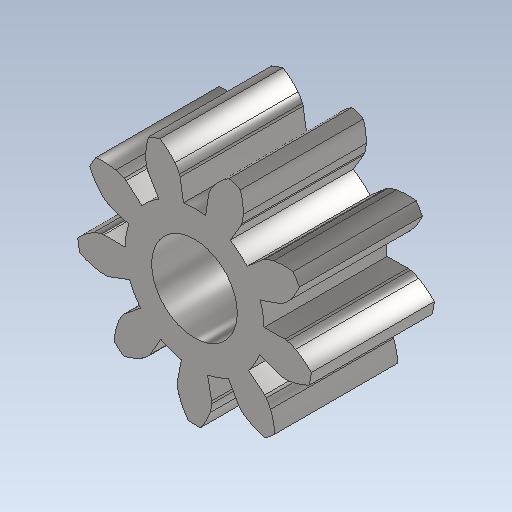
# Autodesk Inventor part: m1歯数9ギアd4t5
Saved by Autodesk Inventor 2020.2 (Build 242310000, 310)
## iProperties
Created: 2020-03-15
Part Number: m1歯数9ギアd4t5
Material: 鋼、炭素鋼
Document SubType Name: Modeling
Designer: aoyam
Density: 7.85 g/cm^3
Appearance: 半つや出し
Mass: 2.14409 g
Surface Area: 5.02952 cm^2
Volume: 0.273133 cm^3
Author: aoyam
Autodesk Inventor part; units mm, degrees
ref_plane "YZ Plane" through (0, 0, 0) normal (1, 0, 0) x (0, 1, 0)
ref_plane "XZ Plane" through (0, 0, 0) normal (0, 1, 0) x (-1, 0, 0)
ref_plane "XY Plane" through (0, 0, 0) normal (0, 0, 1) x (1, 0, 0)
sketch "スケッチ1" plane through (0, 0, 0) normal (0, 0, 1) x (1, 0, 0)
  arc A0 (1.9666, 4.772) -> (1.9302, 4.6607) centre (2.4755, 4.5436) ccw
  arc A1 (2.1768, 5.1207) -> (1.9666, 4.772) centre (3.3978, 4.1472) ccw
  arc A2 (2.8705, 5.7442) -> (2.1768, 5.1207) centre (4.3759, 3.3715) ccw
  arc A3 (0.5859, 4.6607) -> (0.5494, 4.772) centre (0.0406, 4.5436) ccw
  arc A4 (0.5494, 4.772) -> (0.3392, 5.1207) centre (-0.8817, 4.1472) ccw
  arc A5 (0.3392, 5.1207) -> (-0.3545, 5.7442) centre (-1.8598, 3.3715) ccw
  arc A6 (1.7746, 3.6946) -> (0.7414, 3.6946) centre (1.258, 0.4859) ccw
  arc A7 (-0.3545, 5.7442) -> (-0.8867, 5.5505) centre (1.258, 0.4859) ccw
  line L0 (1.7746, 3.6946) -> (1.9302, 4.6607)
  line L1 (0.7414, 3.6946) -> (0.5859, 4.6607)
  line L2 (-1.2002, 2.6118) -> (-1.9404, 3.2519)
  arc A8 (-1.9404, 3.2519) -> (-2.0398, 3.3137) centre (-2.2829, 2.8117) ccw
  arc A9 (-2.0398, 3.3137) -> (-2.425, 3.4458) centre (-2.7345, 1.9152) ccw
  arc A10 (-2.425, 3.4458) -> (-3.3572, 3.4775) centre (-2.9852, 0.6922) ccw
  arc A11 (-3.3572, 3.4775) -> (-3.6404, 2.987) centre (1.258, 0.4859) ccw
  arc A12 (-0.4087, 3.2759) -> (-1.2002, 2.6118) centre (1.258, 0.4859) ccw
  arc A13 (-0.9542, 4.2247) -> (-0.9106, 4.116) centre (-0.4176, 4.3769) ccw
  line L3 (-0.4087, 3.2759) -> (-0.9106, 4.116)
  arc A14 (-1.0174, 4.627) -> (-0.9542, 4.2247) centre (0.5437, 4.666) ccw
  arc A15 (-0.8867, 5.5505) -> (-1.0174, 4.627) centre (1.7917, 4.7005) ccw
  line L4 (-1.9916, 0.5343) -> (-2.9701, 0.5489)
  arc A16 (-2.9701, 0.5489) -> (-3.086, 0.5323) centre (-2.9495, -0.0085) ccw
  arc A17 (-3.086, 0.5323) -> (-3.466, 0.3859) centre (-2.7192, -0.9856) ccw
  arc A18 (-3.466, 0.3859) -> (-4.2004, -0.189) centre (-2.1251, -2.0836) ccw
  arc A19 (-4.2004, -0.189) -> (-4.102, -0.7468) centre (1.258, 0.4859) ccw
  arc A20 (-1.8122, 1.5518) -> (-1.9916, 0.5343) centre (1.258, 0.4859) ccw
  arc A21 (-2.8399, 1.928) -> (-2.7367, 1.8728) centre (-2.5267, 2.3895) ccw
  line L5 (-1.8122, 1.5518) -> (-2.7367, 1.8728)
  arc A22 (-3.1469, 2.1955) -> (-2.8399, 1.928) centre (-1.9761, 3.2289) ccw
  arc A23 (-3.6404, 2.987) -> (-3.1469, 2.1955) centre (-1.0423, 4.0575) ccw
  line L6 (-1.2625, -1.5659) -> (-2.0214, -2.1837)
  arc A24 (-2.0214, -2.1837) -> (-2.0995, -2.2708) centre (-1.6474, -2.5974) ccw
  arc A25 (-2.0995, -2.2708) -> (-2.2965, -2.6273) centre (-0.8429, -3.1978) ccw
  arc A26 (-2.2965, -2.6273) -> (-2.4895, -3.5398) centre (0.318, -3.6571) ccw
  arc A27 (-2.4895, -3.5398) -> (-2.0557, -3.9038) centre (1.258, 0.4859) ccw
  arc A28 (-1.7791, -0.6711) -> (-1.2625, -1.5659) centre (1.258, 0.4859) ccw
  arc A29 (-2.8081, -1.0435) -> (-2.6936, -1.0195) centre (-2.8648, -0.4887) ccw
  line L7 (-1.7791, -0.6711) -> (-2.6936, -1.0195)
  arc A30 (-3.2153, -1.0359) -> (-2.8081, -1.0435) centre (-2.9826, 0.5083) ccw
  arc A31 (-4.102, -0.7468) -> (-3.2153, -1.0359) centre (-2.7999, 1.7432) ccw
  line L8 (0.646, -2.706) -> (0.4618, -3.6671)
  arc A32 (0.4618, -3.6671) -> (0.458, -3.7841) centre (1.0142, -3.7436) ccw
  arc A33 (0.458, -3.7841) -> (0.5362, -4.1837) centre (2.0165, -3.6865) ccw
  arc A34 (0.5362, -4.1837) -> (0.9748, -5.0068) centre (3.201, -3.2921) ccw
  arc A35 (0.9748, -5.0068) -> (1.5412, -5.0068) centre (1.258, 0.4859) ccw
  arc A36 (-0.3248, -2.3526) -> (0.646, -2.706) centre (1.258, 0.4859) ccw
  arc A37 (-0.8737, -3.2994) -> (-0.8015, -3.2073) centre (-1.2738, -2.9108) ccw
  line L9 (-0.3248, -2.3526) -> (-0.8015, -3.2073)
  arc A38 (-1.1906, -3.5552) -> (-0.8737, -3.2994) centre (-2.0049, -2.2228) ccw
  arc A39 (-2.0557, -3.9038) -> (-1.1906, -3.5552) centre (-2.6587, -1.1593) ccw
  line L10 (2.8409, -2.3526) -> (3.3175, -3.2073)
  arc A40 (3.3175, -3.2073) -> (3.3898, -3.2994) centre (3.7899, -2.9108) ccw
  arc A41 (3.3898, -3.2994) -> (3.7066, -3.5552) centre (4.521, -2.2228) ccw
  arc A42 (3.7066, -3.5552) -> (4.5717, -3.9038) centre (5.1748, -1.1593) ccw
  arc A43 (4.5717, -3.9038) -> (5.0056, -3.5398) centre (1.258, 0.4859) ccw
  arc A44 (1.87, -2.706) -> (2.8409, -2.3526) centre (1.258, 0.4859) ccw
  arc A45 (2.0581, -3.7841) -> (2.0543, -3.6671) centre (1.5018, -3.7436) ccw
  line L11 (1.87, -2.706) -> (2.0543, -3.6671)
  arc A46 (1.9799, -4.1837) -> (2.0581, -3.7841) centre (0.4996, -3.6865) ccw
  arc A47 (1.5412, -5.0068) -> (1.9799, -4.1837) centre (-0.6849, -3.2921) ccw
  line L12 (4.2951, -0.6711) -> (5.2096, -1.0195)
  arc A48 (5.2096, -1.0195) -> (5.3242, -1.0435) centre (5.3809, -0.4887) ccw
  arc A49 (5.3242, -1.0435) -> (5.7314, -1.0359) centre (5.4987, 0.5083) ccw
  arc A50 (5.7314, -1.0359) -> (6.6181, -0.7468) centre (5.316, 1.7432) ccw
  arc A51 (6.6181, -0.7468) -> (6.7165, -0.189) centre (1.258, 0.4859) ccw
  arc A52 (3.7785, -1.5659) -> (4.2951, -0.6711) centre (1.258, 0.4859) ccw
  arc A53 (4.6156, -2.2708) -> (4.5375, -2.1837) centre (4.1634, -2.5974) ccw
  line L13 (3.7785, -1.5659) -> (4.5375, -2.1837)
  arc A54 (4.8126, -2.6273) -> (4.6156, -2.2708) centre (3.359, -3.1978) ccw
  arc A55 (5.0056, -3.5398) -> (4.8126, -2.6273) centre (2.1981, -3.6571) ccw
  line L14 (4.3283, 1.5518) -> (5.2528, 1.8728)
  arc A56 (5.2528, 1.8728) -> (5.356, 1.928) centre (5.0428, 2.3895) ccw
  arc A57 (5.356, 1.928) -> (5.663, 2.1955) centre (4.4922, 3.2289) ccw
  arc A58 (5.663, 2.1955) -> (6.1565, 2.987) centre (3.5584, 4.0575) ccw
  arc A59 (6.1565, 2.987) -> (5.8733, 3.4775) centre (1.258, 0.4859) ccw
  arc A60 (4.5077, 0.5343) -> (4.3283, 1.5518) centre (1.258, 0.4859) ccw
  arc A61 (5.6021, 0.5323) -> (5.4862, 0.5489) centre (5.4656, -0.0085) ccw
  line L15 (4.5077, 0.5343) -> (5.4862, 0.5489)
  arc A62 (5.982, 0.3859) -> (5.6021, 0.5323) centre (5.2353, -0.9856) ccw
  arc A63 (6.7165, -0.189) -> (5.982, 0.3859) centre (4.6412, -2.0836) ccw
  line L16 (2.9248, 3.2759) -> (3.4267, 4.116)
  arc A64 (3.4267, 4.116) -> (3.4703, 4.2247) centre (2.9337, 4.3769) ccw
  arc A65 (3.4703, 4.2247) -> (3.5334, 4.627) centre (1.9724, 4.666) ccw
  arc A66 (3.5334, 4.627) -> (3.4028, 5.5505) centre (0.7244, 4.7005) ccw
  arc A67 (3.4028, 5.5505) -> (2.8705, 5.7442) centre (1.258, 0.4859) ccw
  arc A68 (3.7163, 2.6118) -> (2.9248, 3.2759) centre (1.258, 0.4859) ccw
  arc A69 (4.5559, 3.3137) -> (4.4565, 3.2519) centre (4.799, 2.8117) ccw
  line L17 (3.7163, 2.6118) -> (4.4565, 3.2519)
  arc A70 (4.9411, 3.4458) -> (4.5559, 3.3137) centre (5.2506, 1.9152) ccw
  arc A71 (5.8733, 3.4775) -> (4.9411, 3.4458) centre (5.5013, 0.6922) ccw
  circle A72 centre (1.258, 0.4859) radius 2
  point P0 (0, 0)
  point P1 (3.7163, 2.6118)
  point P2 (2.9248, 3.2759)
  point P3 (3.4678, 4.2162)
  point P4 (3.5333, 4.6228)
  point P5 (3.4028, 5.5505)
  point P6 (2.8705, 5.7442)
  point P7 (2.1742, 5.1175)
  point P8 (1.9631, 4.7639)
  point P9 (1.7746, 3.6946)
  point P10 (0.7414, 3.6946)
  point P11 (0.5859, 4.6607)
  point P12 (0.553, 4.7639)
  point P13 (0.3418, 5.1175)
  point P14 (-0.3545, 5.7442)
  point P15 (-0.8867, 5.5505)
  point P16 (-1.0172, 4.6228)
  point P17 (-0.9517, 4.2162)
  point P18 (-1.2002, 2.6118)
  point P19 (-2.0319, 3.3098)
  point P20 (-2.4209, 3.445)
  point P21 (-3.3572, 3.4775)
  point P22 (-3.6404, 2.987)
  point P23 (-3.1441, 2.1924)
  point P24 (-2.8326, 1.9231)
  point P25 (-1.8122, 1.5518)
  point P26 (-1.9916, 0.5343)
  point P27 (-2.9701, 0.5489)
  point P28 (-3.0774, 0.5344)
  point P29 (-3.4623, 0.3879)
  point P30 (-4.2004, -0.189)
  point P31 (-4.102, -0.7468)
  point P32 (-3.2111, -1.0365)
  point P33 (-2.7994, -1.0426)
  point P34 (-1.7791, -0.6711)
  point P35 (-1.2625, -1.5659)
  point P36 (-2.0214, -2.1837)
  point P37 (-2.0943, -2.2638)
  point P38 (-2.2949, -2.6234)
  point P39 (-2.4895, -3.5398)
  point P40 (-2.0557, -3.9038)
  point P41 (-1.187, -3.5531)
  point P42 (-0.8677, -3.293)
  point P43 (-0.8015, -3.2073)
  point P44 (-0.3248, -2.3526)
  point P45 (0.4574, -3.7753)
  point P46 (0.5349, -4.1798)
  point P47 (0.9748, -5.0068)
  point P48 (1.5412, -5.0068)
  point P49 (1.9812, -4.1798)
  point P50 (2.0587, -3.7753)
  point P51 (2.0543, -3.6671)
  point P52 (1.87, -2.706)
  point P53 (2.8409, -2.3526)
  point P54 (3.3175, -3.2073)
  point P55 (3.3838, -3.293)
  point P56 (3.7031, -3.5531)
  point P57 (4.5717, -3.9038)
  point P58 (5.0056, -3.5398)
  point P59 (4.811, -2.6234)
  point P60 (4.6104, -2.2638)
  point P61 (4.5375, -2.1837)
  point P62 (5.3155, -1.0426)
  point P63 (5.7272, -1.0365)
  point P64 (6.6181, -0.7468)
  point P65 (6.7165, -0.189)
  point P66 (5.9784, 0.3879)
  point P67 (5.5935, 0.5344)
  point P68 (5.3487, 1.9231)
  point P69 (5.6602, 2.1924)
  point P70 (6.1565, 2.987)
  point P71 (5.8733, 3.4775)
  point P72 (4.937, 3.445)
  point P73 (4.548, 3.3098)
  point P74 (4.4565, 3.2519)
  dimension "d2" = 360
  dimension "d4" = 4
  constraints: 144 point on circle, 73 centre point, 36 end point, 2 coincident, 359 other
  measures "d4" diameter of A72
extrude "押し出し1" add sketch "スケッチ1" along normal blind 5.75
